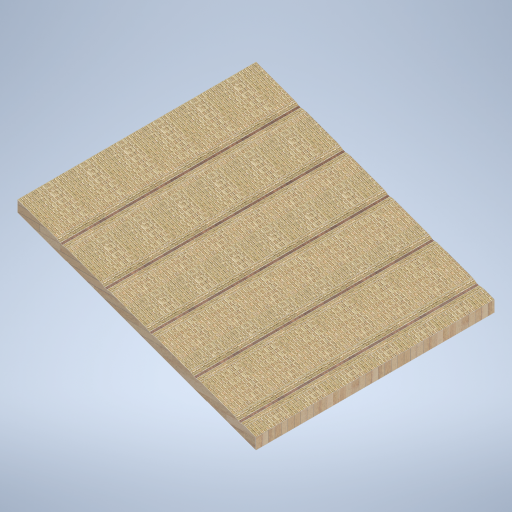
# Autodesk Inventor part: side_curve_panel_01
Saved by Autodesk Inventor 2024.2 (Build 282272000, 272)
## iProperties
Created: 2024-05-24
Part Number: side_curve_panel_01
Material: Wood (Maple)
Document SubType Name: Modeling
Designer: LOSTER_1
Density: 0.67 g/cm^3
Appearance: Natural Maple - Glossy Dark Tint
Author: LOSTER_1
Autodesk Inventor part; units mm, degrees
ref_plane "XZ Plane" through (0, 0, 0) normal (0, 1, 0) x (-1, 0, 0)
ref_plane "XY Plane" through (0, 0, 0) normal (0, 0, 1) x (1, 0, 0)
sketch "Sketch1" plane through (0, 0, 0) normal (1, 0, 0) x (0, 1, 0)
  line L0 (-50, 1055.5) -> (50, 1055.5)
  line L1 (50, 1055.5) -> (50, -1055.5)
  line L2 (50, -1055.5) -> (-50, -1055.5)
  line L3 (-50, -1055.5) -> (-50, 1055.5)
  line L4 (-50, 1055.5) -> (50, -1055.5) construction
  line L5 (50, 1055.5) -> (-50, -1055.5) construction
  point P0 (0, 0)
  dimension "d0" = 100
  dimension "d1" = 2111
  constraints: 12 end point, 2 midpoint, 2 parallel, 1 horizontal, 1 perpendicular
  measures "d0" distance of L1.end L2.end
  measures "d1" distance of L0.end L1.end
ref_plane "Work Plane2" through (2109, 0, 0) normal (1, 0, 0) x (0, 1, 0)
ref_plane "Work Plane1" through (0, 0, 0) normal (1, 0, 0) x (0, 1, 0)
sketch "Sketch3" plane through (2109, 0, 0) normal (1, 0, 0) x (0, 1, 0)
  line L0 (-50, 1055.5) -> (50, 1055.5) projected
  point P0 (0, 0)
ref_plane "Work Plane3" through (0, -50, 1055.5) normal (0, 0, -1) x (0, 1, 0)
sketch "Sketch4" plane through (0, -50, 1055.5) normal (0, 0, -1) x (0, 1, 0)
  line L0 (0, 2109) -> (100, 2109) projected
  line L1 (100, 0) -> (-667.6132, 2109)
  line L2 (100, 0) -> (2344.3509, 0) construction
  line L3 (0, 0) -> (-767.6132, 2109)
  line L4 (0, 0) -> (2244.3509, 0) construction
  line L5 (-667.6132, 2109) -> (-767.6132, 2109)
  line L6 (100, 0) -> (0, 0)
  point P0 (50, 0)
  dimension "d4" = 110
  dimension "d5" = 110
  constraints: 12 end point, 3 horizontal, 2 equal length, 1 collinear
  measures "d4" angle of L2 L1
  measures "d5" angle of L4 L3
extrude "Extrusion1" add sketch "Sketch4" along normal blind 2111
sketch "Sketch5" plane through (0, -50, -1055.5) normal (0, 0, -1) x (-1, 0, 0)
  line L0 (0, 100) -> (-2109, -667.6132) projected
  line L1 (0, 100) -> (-375.877, -36.8081)
  line L2 (-375.877, -36.8081) -> (-375.877, -46.8081)
  line L3 (-375.877, -46.8081) -> (-394.6709, -53.6485)
  line L4 (-394.6709, -53.6485) -> (-394.6709, -43.6485)
  line L5 (-394.6709, -43.6485) -> (-770.5479, -180.4565)
  line L6 (-770.5479, -180.4565) -> (-770.5479, -190.4565)
  line L7 (-770.5479, -190.4565) -> (-789.3418, -197.2969)
  line L8 (-789.3418, -197.2969) -> (-789.3418, -187.2969)
  line L9 (-789.3418, -187.2969) -> (-1165.2188, -324.105)
  line L10 (-1165.2188, -324.105) -> (-1165.2188, -334.105)
  line L11 (-1165.2188, -334.105) -> (-1184.0127, -340.9454)
  line L12 (-1184.0127, -340.9454) -> (-1184.0127, -330.9454)
  line L13 (-1184.0127, -330.9454) -> (-1559.8898, -467.7534)
  line L14 (-1559.8898, -467.7534) -> (-1558.7864, -477.3518)
  line L15 (-1558.7864, -477.3518) -> (-1577.5802, -484.1922)
  line L16 (-1577.5802, -484.1922) -> (-1577.5802, -474.1922)
  line L17 (-1577.5802, -474.1922) -> (-1953.4573, -611.0003)
  line L18 (-1953.4573, -611.0003) -> (-1953.4573, -621.0003)
  line L19 (-1953.4573, -621.0003) -> (-1972.2511, -627.8407)
  line L20 (-1972.2511, -627.8407) -> (-1972.2511, -617.8407)
  line L21 (-1972.2511, -617.8407) -> (-375.877, -36.8081)
  point P0 (0, 50)
  dimension "d8" = 400
  dimension "d9" = 10
  dimension "d10" = 20
  dimension "d11" = 400
  dimension "d12" = 20
  dimension "d13" = 400
  dimension "d14" = 20
  dimension "d15" = 400
  dimension "d16" = 20
  dimension "d17" = 400
  dimension "d18" = 20
  constraints: 42 end point, 9 parallel, 6 point on line, 2 vertical, 1 collinear, 11 other
  measures "d8" distance of L1.start L1.end
  measures "d9" distance of L1.end L2.end
  measures "d10" distance of L2.end L3.end
  measures "d11" distance of L4.end L5.end
  measures "d12" distance of L6.end L7.end
  measures "d13" distance of L8.end L9.end
  measures "d14" distance of L10.end L11.end
  measures "d15" distance of L12.end L13.end
  measures "d16" distance of L14.end L15.end
  measures "d17" distance of L16.end L17.end
  measures "d18" distance of L18.end L19.end
extrude "Extrusion2" cut sketch "Sketch5" against normal through all
fillet "Fillet1" radius 100 10 edges at (1972.2511, -667.8407, 0) (1953.4573, -661.0003, 0) (1577.5802, -524.1922, 0) (1559.8898, -517.7534, 0) (1184.0127, -380.9454, 0) (1165.2188, -374.105, 0) (789.3418, -237.2969, 0) (770.5479, -230.4565, 0) (394.6709, -93.6485, 0) (375.877, -86.8081, 0)
body "Solid1"
